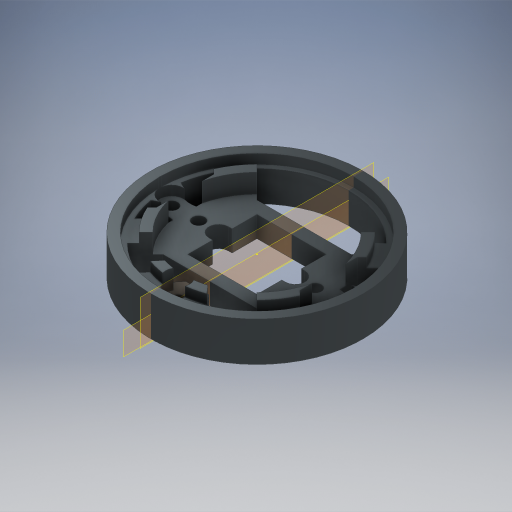
# Autodesk Inventor part: omv_centre
Saved by Autodesk Inventor 2023 (Build 270158000, 158)
## iProperties
Created: 2024-12-20
Part Number: omv_centre
Material: Типовые
Document SubType Name: Modeling
Designer: Ivan
Density: 1 g/cm^3
Appearance: Чугун серый
Mass: 9.16198 g
Surface Area: 75.1348 cm^2
Volume: 9.16198 cm^3
Author: Ivan
Autodesk Inventor part; units mm, degrees
ref_plane "XZ Plane" through (0, 0, 0) normal (0, 1, 0) x (-1, 0, 0)
ref_plane "XY Plane" through (0, 0, 0) normal (0, 0, 1) x (1, 0, 0)
sketch "Эскиз3" plane through (0, 0, 0) normal (0, 1, 0) x (-1, 0, 0)
  circle A0 centre (0, 0) radius 7
  arc A1 (-1.5597, 7.5914) -> (1.5597, 7.5914) centre (0, 0) ccw
  line L0 (1.4, 8.3) -> (1.4, 7.7873)
  arc A2 (1.4, 7.7873) -> (1.5597, 7.5914) centre (1.6, 7.7873) ccw
  arc A3 (1.4, 8.3) -> (1.2, 8.5) centre (1.2, 8.3) ccw
  line L1 (-1.2, 8.5) -> (1.2, 8.5)
  arc A4 (-1.2, 8.5) -> (-1.4, 8.3) centre (-1.2, 8.3) ccw
  line L2 (-1.4, 7.7873) -> (-1.4, 8.3)
  arc A5 (-1.5597, 7.5914) -> (-1.4, 7.7873) centre (-1.6, 7.7873) ccw
  line L3 (8.5, 7.5) -> (8.5, 1.9)
  arc A6 (8.5, 7.5) -> (7.5, 8.5) centre (7.5, 7.5) ccw
  line L4 (1.6, 8.5) -> (7.5, 8.5)
  line L5 (8.5, -1.9) -> (8.5, -7.5)
  arc A7 (7.5, -8.5) -> (8.5, -7.5) centre (7.5, -7.5) ccw
  line L6 (7.5, -8.5) -> (-7.5, -8.5)
  arc A8 (-8.5, -7.5) -> (-7.5, -8.5) centre (-7.5, -7.5) ccw
  line L7 (-8.5, -7.5) -> (-8.5, -1.9)
  line L8 (-7.5, 8.5) -> (-1.6, 8.5)
  arc A9 (-7.5, 8.5) -> (-8.5, 7.5) centre (-7.5, 7.5) ccw
  line L9 (-8.5, 1.9) -> (-8.5, 7.5)
  line L10 (-1.2, 8.5) -> (-1.6, 8.5)
  line L11 (1.6, 8.5) -> (1.2, 8.5)
  circle A10 centre (15.24, 0) radius 1.5
  circle A11 centre (-15.24, 0) radius 1.5
  arc A12 (-10, 1.9) -> (-10, -1.9) centre (-10, 0) ccw
  arc A13 (10, -1.9) -> (10, 1.9) centre (10, 0) ccw
  line L12 (8.5, 1.9) -> (10, 1.9)
  line L13 (10, -1.9) -> (8.5, -1.9)
  line L14 (-10, 1.9) -> (-8.5, 1.9)
  line L15 (-8.5, -1.9) -> (-10, -1.9)
  constraints: 32 end point, 22 point on circle, 14 centre point
sketch "Эскиз4" plane through (0, 0, 0) normal (0, 1, 0) x (-1, 0, 0)
  circle A0 centre (0, 0) radius 29
  circle A1 centre (0, 0) radius 26.45
  circle A2 centre (0, 0) radius 23.95
  circle A3 centre (0, 0) radius 31.5
  line L0 (-9.05, 2.55) -> (-9.05, 9.05)
  line L1 (-9.05, 9.05) -> (9.05, 9.05)
  line L2 (9.05, 9.05) -> (9.05, 2.55)
  line L3 (-9.05, -2.55) -> (-9.05, -9.05)
  line L4 (-9.05, -9.05) -> (9.05, -9.05)
  line L5 (9.05, -9.05) -> (9.05, -2.55)
  line L6 (-1.2, 8.5) -> (1.2, 8.5) projected
  line L7 (0, 8.5) -> (0, 9.05) construction
  line L8 (8.5, 7.5) -> (8.5, 1.9) projected
  line L9 (-8.5, 1.9) -> (-8.5, 7.5) projected
  line L10 (7.5, -8.5) -> (-7.5, -8.5) projected
  line L11 (8.5, 1.9) -> (10, 1.9) projected
  line L12 (9.05, 2.55) -> (10, 2.55)
  line L13 (9.05, -2.55) -> (10, -2.55)
  line L14 (-9.05, -2.55) -> (-10, -2.55)
  line L15 (-9.05, 2.55) -> (-10, 2.55)
  line L16 (10, 1.9) -> (10, 2.55) construction
  line L17 (10, 2.55) -> (10, -2.55) construction
  line L18 (-10, 2.55) -> (-10, -2.55) construction
  arc A4 (10, -2.55) -> (10, 2.55) centre (10, 0) ccw
  arc A5 (-10, 2.55) -> (-10, -2.55) centre (-10, 0) ccw
  circle A6 centre (-15.24, 0) radius 1.5 construction
  circle A7 centre (15.24, 0) radius 1.5 construction
  circle A8 centre (-15.24, 0) radius 1.6
  circle A9 centre (15.24, 0) radius 1.6
  line L19 (-9.05, 9.05) -> (-16.9352, 16.9352)
  line L20 (-9.05, -9.05) -> (-16.9352, -16.9352)
  line L21 (9.05, -9.05) -> (16.9352, -16.9352)
  line L22 (9.05, 9.05) -> (16.9352, 16.9352)
  line L23 (44.1, 0) -> (-44.1, 0) projected
  circle A10 centre (15.24, 0) radius 3.5 construction
  circle A11 centre (-15.24, 0) radius 3.5 construction
  line L24 (-18.74, 7.5) -> (-18.74, -7.5)
  line L25 (18.74, 7.5) -> (18.74, -7.5)
  line L26 (-18.74, 7.5) -> (-21.5955, 10.3555)
  line L27 (-18.74, -7.5) -> (-21.5955, -10.3555)
  line L28 (18.74, 7.5) -> (21.5955, 10.3555)
  line L29 (18.74, -7.5) -> (21.5955, -10.3555)
  line L30 (-12.28, 12.28) -> (12.28, 12.28)
  line L31 (-12.28, -12.28) -> (12.28, -12.28)
  point P0 (-16.84, 0)
  point P1 (16.84, 0)
  point P2 (18.74, 0)
  point P3 (-18.74, 0)
  dimension "d11" = 3.2
  dimension "d16" = 7
  dimension "d1" = 58
  dimension "d3" = 2.55
  dimension "d4" = 2.5
  dimension "d5" = 2.5
  dimension "d6" = 0.55
  dimension "d7" = 0.55
  dimension "d8" = 0.55
  dimension "d9" = 0.65
  dimension "d10" = 0.55
  dimension "d13" = 135
  dimension "d14" = 135
  dimension "d17" = 135
  dimension "d18" = 15
  dimension "d19" = 9.69
  dimension "d20" = 3.23
  dimension "d21" = 3.23
  constraints: 52 end point, 11 perpendicular, 8 coincident, 7 equal length, 6 midpoint, 6 point on line, 6 vertical, 5 centre point, 5 parallel, 4 horizontal alignment, 4 point on circle, 2 collinear, 2 horizontal, 18 other
  measures "d1" diameter of A0
  measures "d3" radial gap between concentric circles of A0 A1
  measures "d5" radial gap between concentric circles of A3 A0
  measures "d6" distance between parallel lines of L1 L6
  measures "d7" distance between parallel lines of L2 L8
  measures "d8" distance between parallel lines of L4 L10
  measures "d9" distance from line of L2.end L11
  measures "d10" distance between parallel lines of L9 L0
  measures "d13" angle of L22 L1
  measures "d14" angle of L19 L1
  measures "d17" angle of L28 L25
  measures "d18" distance of L24.start L24.end
  measures "d19" distance from line of L0 point (-18.74, 0)
  measures "d20" distance between parallel lines of L1 L30
  measures "d21" distance between parallel lines of L4 L31
extrude "Выдавливание1" add sketch "Эскиз4" along normal blind 5.5 contours L23 A3 A0 | A0 L23 A3 | L23 A2 A1 | A1 L23 A2 | L28 L25 L23 A9 A4 L12 L2 L22 A2 | A2 L21 L5 L13 A4 L23 A9 L25 L29 | A2 L19 L0 L15 A5 L23 A8 L24 L26 | L27 L24 L23 A8 A5 L14 L3 L20 A2 | L22 L1 L19 L30 | L31 L20 L4 L21
extrude "Выдавливание2" add sketch "Эскиз4" along normal blind 3.5 contours L23 A1 A0 | A0 L23 A1
chamfer "Фаска1" distance 4 angle 45 1 edges at (31.5, 0, 0)
sketch "Эскиз6" plane through (0, 0, 0) normal (0, -1, 0) x (1, 0, 0)
  circle A0 centre (-0.1305, 20.6127) radius 2.1 projected
  point P0 (0, 0)
sketch "Эскиз7" plane through (0, 0, 0) normal (0, -1, 0) x (1, 0, 0)
  circle A0 centre (-0.1305, 20.6127) radius 2.1 construction
  circle A1 centre (-0.1305, 20.6127) radius 1.6
  circle A2 centre (0, 0) radius 23.95 projected
  arc A3 (16.9352, 16.9352) -> (-16.9352, 16.9352) centre (0, 0) ccw projected
  line L0 (-8.9159, 22.2286) -> (-3.9, 17.2127)
  line L1 (-3.9, 17.2127) -> (3.9, 17.2127)
  line L2 (3.9, 17.2127) -> (8.9159, 22.2286)
  circle A4 centre (-0.1305, 20.6127) radius 3.4 construction
  point P0 (8.9159, 22.2286)
  dimension "d33" = 3.2
  dimension "d34" = 135
  dimension "d35" = 135
  dimension "d36" = 6.8
  dimension "d37" = 7.8
  constraints: 6 end point, 2 centre point, 2 coincident, 2 point on circle, 1 horizontal, 1 perpendicular, 1 tangent
  measures "d33" diameter of A1
  measures "d34" angle of L0 L1
  measures "d35" angle of L2 L1
  measures "d36" diameter of A4
  measures "d37" distance of L0.end L1.end
extrude "Выдавливание3" add sketch "Эскиз7" against normal up to surface (5.5 mm away) contours L2 L1 L0 A2 picked at (-5.7854, 20.9857)
sketch "Эскиз8" plane through (0, 0, 0) normal (0, -1, 0) x (1, 0, 0)
  circle A0 centre (14.6021, 5.1056) radius 2.1 projected
  circle A1 centre (-14.8609, 5.1034) radius 2.1 projected
  point P0 (0, 0)
sketch "Эскиз9" plane through (0, 0, 0) normal (0, -1, 0) x (1, 0, 0)
  circle A0 centre (-14.8609, 5.1034) radius 1.397 projected
  circle A1 centre (14.6031, 5.1142) radius 1.397 projected
  point P0 (0, 0)
sketch "Эскиз11" plane through (0, 0, 0) normal (0, -1, 0) x (1, 0, 0)
  circle A0 centre (15.24, 0) radius 1.6 projected
  circle A1 centre (15.24, 0) radius 3
  point P0 (0, 0)
  dimension "d44" = 6
  constraints: 1 centre point, 1 coincident
  measures "d44" diameter of A1
sketch "Эскиз12" plane through (0, 0, 0) normal (0, -1, 0) x (1, 0, 0)
  circle A0 centre (22.0195, 0) radius 2 projected
  circle A1 centre (27.6855, 0) radius 1.6
  point P0 (0, 0)
  dimension "d50" = 3.2
  dimension "d51" = 5.666
  constraints: 1 centre point
  measures "d50" diameter of A1
  measures "d51" distance of A1.centre A0.centre
sketch "Эскиз13" plane through (0, 0, 0) normal (0, -1, 0) x (1, 0, 0)
  circle A0 centre (22.15, 0.1589) radius 1.6
  circle A1 centre (22.15, 0.1589) radius 3.1 construction
  arc A2 (21.5955, -10.3555) -> (21.5955, 10.3555) centre (0, 0) ccw projected
  line L0 (18.74, 7.5) -> (18.74, -7.5) projected
  arc A3 (21.5955, -10.3555) -> (21.5955, 10.3555) centre (0, 0) ccw projected
  line L1 (18.74, 7.5) -> (18.74, -7.5) projected
  line L2 (21.5955, 10.3555) -> (18.74, 7.5) projected
  line L3 (18.74, -7.5) -> (21.5955, -10.3555) projected
  arc A4 (18.74, 3.2133) -> (23.5905, 4.1342) centre (20.1678, 8.9278) ccw
  arc A5 (23.6473, -3.7958) -> (18.74, -2.8941) centre (20.1678, -8.9278) ccw
  line L4 (0, 44.1) -> (0, -44.1) projected
  point P0 (11.24, 0)
  point P1 (18.74, -2.8941)
  point P2 (23.6473, -3.7958)
  point P3 (23.5905, 4.1342)
  point P4 (18.74, 3.2133)
  dimension "d45" = 3.2
  dimension "d46" = 6.2
  dimension "d49" = 22.15
  constraints: 6 point on circle, 4 centre point, 4 point on line, 3 coincident, 2 midpoint, 2 tangent
  measures "d45" diameter of A0
  measures "d46" diameter of A1
  measures "d49" distance from line of L4 point (22.15, 0.159)
extrude "Выдавливание5" add sketch "Эскиз13" against normal up to surface (5.5 mm away) contours A5 L0 A4 A2
ref_plane "РабПлоскость1" through (0, 0, 9.05) normal (1, 0, 0) x (0, 0, -1)
mirror "Зеркальное отражение2" about plane through (0, 0, 9.05) normal (1, 0, 0) of "Выдавливание5"
sketch "Эскиз14" plane through (0, 5.5, 0) normal (0, 1, 0) x (1, 0, 0)
  line L0 (3.9, -17.2127) -> (8.9159, -22.2286) projected
  line L1 (-8.9159, -22.2286) -> (-3.9, -17.2127) projected
  arc A0 (-16.9352, -16.9352) -> (-8.9159, -22.2286) centre (0, 0) ccw projected
  arc A1 (8.9159, -22.2286) -> (16.9352, -16.9352) centre (0, 0) ccw projected
  circle A2 centre (0, 0) radius 23.95
  line L2 (-8.9159, -22.2286) -> (-3.1305, -15.4166)
  line L3 (-3.1305, -15.4166) -> (2.8695, -15.4166)
  line L4 (3.9, -17.2127) -> (8.9159, -22.2286) projected
  line L5 (2.8695, -15.4166) -> (8.9159, -22.2286)
  line L6 (-3.9, -17.2127) -> (3.9, -17.2127) projected
  line L7 (-3.9, -17.2127) -> (3.9, -17.2127)
  line L8 (-8.9159, -22.2286) -> (-3.9, -17.2127) projected
  line L9 (-3.9, -17.2127) -> (3.9, -17.2127) projected
  line L10 (-3.9, -17.2127) -> (3.9, -17.2127)
  constraints: 10 end point, 3 point on circle, 1 centre point, 1 collinear, 1 horizontal, 2 other
extrude "Выдавливание6" add sketch "Эскиз14" against normal up to surface (5.5 mm away) contours L6 L1 L2 L3 L5 L0
sketch "Эскиз15" plane through (0, 5.5, 0) normal (0, 1, 0) x (1, 0, 0)
  point P0 (0, 0)
sketch "Эскиз16" plane through (0, 5.5, 0) normal (0, 1, 0) x (1, 0, 0)
  circle A0 centre (0, 0) radius 29 projected
  circle A1 centre (0, 0) radius 26.45 projected
extrude "Выдавливание7" add sketch "Эскиз16" against normal up to surface (2 mm away)
sketch "Эскиз17" plane through (0, 5.5, 0) normal (0, 1, 0) x (1, 0, 0)
  circle A0 centre (0, 0) radius 21.75
  circle A1 centre (0, 0) radius 25.25
  circle A2 centre (0, 0) radius 31.5 projected
  arc A3 (-21.5955, 10.3555) -> (-23.6473, 3.7958) centre (0, 0) ccw projected
  line L0 (-21.5955, 10.3555) -> (-18.74, 7.5) projected
  line L1 (-18.74, 7.5) -> (-18.74, 2.8941) projected
  arc A4 (-23.6473, 3.7958) -> (-18.74, 2.8941) centre (-20.1678, 8.9278) ccw projected
  circle A5 centre (-22.15, -0.1589) radius 1.6 projected
  arc A6 (21.5955, -10.3555) -> (23.5905, -4.1342) centre (0, 0) ccw projected
  line L2 (21.5955, -10.3555) -> (18.74, -7.5) projected
  line L3 (18.74, -7.5) -> (18.74, -3.2133) projected
  arc A7 (23.5905, -4.1342) -> (18.74, -3.2133) centre (20.1678, -8.9278) ccw projected
  circle A8 centre (22.15, -0.1589) radius 1.6 projected
  circle A9 centre (-0.1305, -20.6127) radius 1.6 projected
  arc A10 (18.74, 2.8941) -> (23.6473, 3.7958) centre (20.1678, 8.9278) ccw projected
  line L4 (18.74, 2.8941) -> (18.74, 7.5) projected
  line L5 (18.74, 7.5) -> (21.5955, 10.3555) projected
  arc A11 (23.6473, 3.7958) -> (21.5955, 10.3555) centre (0, 0) ccw projected
  arc A12 (-18.74, -3.2133) -> (-23.5905, -4.1342) centre (-20.1678, -8.9278) ccw projected
  line L6 (-18.74, -3.2133) -> (-18.74, -7.5) projected
  line L7 (-18.74, -7.5) -> (-21.5955, -10.3555) projected
  arc A13 (-23.5905, -4.1342) -> (-21.5955, -10.3555) centre (0, 0) ccw projected
  line L8 (-16.9352, -16.9352) -> (-12.28, -12.28) projected
  line L9 (-12.28, -12.28) -> (12.28, -12.28) projected
  line L10 (12.28, -12.28) -> (16.9352, -16.9352) projected
  arc A14 (8.9159, -22.2286) -> (16.9352, -16.9352) centre (0, 0) ccw projected
  line L11 (8.9159, -22.2286) -> (2.8695, -15.4166) projected
  line L12 (2.8695, -15.4166) -> (-3.1305, -15.4166) projected
  line L13 (-3.1305, -15.4166) -> (-8.9159, -22.2286) projected
  arc A15 (-16.9352, -16.9352) -> (-8.9159, -22.2286) centre (0, 0) ccw projected
  circle A16 centre (-15.24, 0) radius 1.6 projected
  circle A17 centre (15.24, 0) radius 1.6 projected
  arc A18 (16.9352, 16.9352) -> (-16.9352, 16.9352) centre (0, 0) ccw projected
  line L14 (16.9352, 16.9352) -> (12.28, 12.28) projected
  line L15 (12.28, 12.28) -> (-12.28, 12.28) projected
  line L16 (-12.28, 12.28) -> (-16.9352, 16.9352) projected
  line L17 (-9.05, -9.05) -> (-9.05, -2.55) projected
  line L18 (-9.05, -2.55) -> (-10, -2.55) projected
  arc A19 (-10, 2.55) -> (-10, -2.55) centre (-10, 0) ccw projected
  line L19 (-10, 2.55) -> (-9.05, 2.55) projected
  line L20 (-9.05, 2.55) -> (-9.05, 9.05) projected
  line L21 (-9.05, 9.05) -> (9.05, 9.05) projected
  line L22 (9.05, 9.05) -> (9.05, 2.55) projected
  line L23 (9.05, 2.55) -> (10, 2.55) projected
  arc A20 (10, -2.55) -> (10, 2.55) centre (10, 0) ccw projected
  line L24 (10, -2.55) -> (9.05, -2.55) projected
  line L25 (9.05, -2.55) -> (9.05, -9.05) projected
  line L26 (9.05, -9.05) -> (-9.05, -9.05) projected
  circle A21 centre (0, 0) radius 27.75
  circle A22 centre (0, 0) radius 19.25
  circle A23 centre (-22.15, -0.1589) radius 3.125
  circle A24 centre (22.15, -0.1589) radius 3.125
  circle A25 centre (-0.1305, -20.6127) radius 1.6 projected
  circle A26 centre (-0.1305, -20.6127) radius 3.125
  point P0 (25.2488, 0.2448)
  point P1 (25.2427, -0.607)
  point P2 (-25.2427, -0.607)
  point P3 (-25.2488, 0.2448)
  point P4 (-18.7899, 7.5499)
  point P5 (-13.6118, 13.6118)
  point P6 (13.6118, 13.6118)
  point P7 (18.7899, 7.5499)
  point P8 (21.8021, 2.9467)
  point P9 (-21.8021, 2.9467)
  point P10 (18.7899, -7.5499)
  point P11 (13.6118, -13.6118)
  point P12 (7.3541, -20.469)
  point P13 (-7.4057, -20.4504)
  point P14 (-13.6118, -13.6118)
  point P15 (-18.7899, -7.5499)
  point P16 (-21.7759, -3.2614)
  point P17 (21.7759, -3.2614)
  point P18 (5.5473, -18.4334)
  point P19 (2.59, -19.075)
  point P20 (-2.8313, -19.0407)
  point P21 (-5.6628, -18.3982)
  point P22 (18.74, 4.4017)
  point P23 (19.0407, 2.8307)
  point P24 (21.1729, 2.8094)
  point P25 (-21.1729, 2.8094)
  point P26 (-19.0407, 2.8307)
  point P27 (-18.74, 4.4017)
  point P28 (19.2268, 0.9458)
  point P29 (19.2112, -1.2215)
  point P30 (-19.2268, 0.9458)
  point P31 (-19.2112, -1.2215)
  point P32 (-18.74, -4.4017)
  point P33 (-18.9894, -3.1567)
  point P34 (-21.1532, -3.1206)
  point P35 (21.1532, -3.1206)
  point P36 (18.9894, -3.1567)
  point P37 (18.74, -4.4017)
  dimension "d56" = 43.5
  dimension "d57" = 50.5
  dimension "d58" = 3.5
  dimension "d59" = 2.5
  dimension "d60" = 2.5
  dimension "d61" = 6.25
  dimension "d62" = 6.25
  dimension "d65" = 6.25
  constraints: 7 coincident, 6 centre point, 2 other
  measures "d56" diameter of A0
  measures "d57" diameter of A1
  measures "d58" radial gap between concentric circles of A1 A0
  measures "d59" radial gap between concentric circles of A21 A1
  measures "d61" diameter of A23
  measures "d62" diameter of A24
  measures "d65" diameter of A26
extrude "Выдавливание8" add sketch "Эскиз17" along normal blind 2.5 contours A10 A11 L5 A0 L14 A18 L16 L0 A3 A4 A23 A1 A24 | A24 A1 A23 A12 A13 L7 A0 L8 A15 L13 A26 L11 A14 L10 L2 A6 A7 | L5 L4 A22 L14 A0 | A0 L10 A22 L3 L2 | L16 A22 L1 L0 A0 | A0 A26 A22 L11 | A0 L13 A22 A26 | L7 L6 A22 L8 A0 | A21
sketch "Эскиз18" plane through (0, 8, 0) normal (0, 1, 0) x (1, 0, 0)
  circle A0 centre (0, 0) radius 19.25 projected
  circle A1 centre (0, 0) radius 21.75 projected
  circle A2 centre (0, 0) radius 27.75 projected
  circle A3 centre (0, 0) radius 25.25
  circle A4 centre (0, 0) radius 27.75 projected
  arc A5 (21.7759, -3.2614) -> (21.8021, 2.9467) centre (22.15, -0.1589) ccw projected
  arc A6 (23.5905, -4.1342) -> (21.7759, -3.2614) centre (20.1678, -8.9278) ccw projected
  arc A7 (13.6118, -13.6118) -> (18.74, -4.4017) centre (0, 0) ccw projected
  arc A8 (2.59, -19.075) -> (5.5473, -18.4334) centre (0, 0) ccw projected
  arc A9 (-5.6628, -18.3982) -> (-2.8313, -19.0407) centre (0, 0) ccw projected
  arc A10 (-21.7759, -3.2614) -> (-23.5905, -4.1342) centre (-20.1678, -8.9278) ccw projected
  arc A11 (-21.8021, 2.9467) -> (-21.7759, -3.2614) centre (-22.15, -0.1589) ccw projected
  arc A12 (-23.6473, 3.7958) -> (-21.8021, 2.9467) centre (-20.1678, 8.9278) ccw projected
  line L0 (-13.6118, 13.6118) -> (-16.9352, 16.9352) projected
  line L1 (16.9352, 16.9352) -> (13.6118, 13.6118) projected
  arc A13 (21.8021, 2.9467) -> (23.6473, 3.7958) centre (20.1678, 8.9278) ccw projected
  arc A14 (21.5955, -10.3555) -> (23.5905, -4.1342) centre (0, 0) ccw projected
  line L2 (21.5955, -10.3555) -> (18.74, -7.5) projected
  line L3 (18.74, -7.5) -> (18.74, -4.4017) projected
  line L4 (13.6118, -13.6118) -> (16.9352, -16.9352) projected
  arc A15 (8.9159, -22.2286) -> (16.9352, -16.9352) centre (0, 0) ccw projected
  line L5 (8.9159, -22.2286) -> (5.5473, -18.4334) projected
  arc A16 (-2.8313, -19.0407) -> (2.59, -19.075) centre (-0.1305, -20.6127) ccw projected
  line L6 (-5.6628, -18.3982) -> (-8.9159, -22.2286) projected
  arc A17 (-16.9352, -16.9352) -> (-8.9159, -22.2286) centre (0, 0) ccw projected
  line L7 (-16.9352, -16.9352) -> (-13.6118, -13.6118) projected
  arc A18 (-18.74, -4.4017) -> (-13.6118, -13.6118) centre (0, 0) ccw projected
  line L8 (-18.74, -4.4017) -> (-18.74, -7.5) projected
  line L9 (-18.74, -7.5) -> (-21.5955, -10.3555) projected
  arc A19 (-23.5905, -4.1342) -> (-21.5955, -10.3555) centre (0, 0) ccw projected
  arc A20 (-21.5955, 10.3555) -> (-23.6473, 3.7958) centre (0, 0) ccw projected
  line L10 (-21.5955, 10.3555) -> (-18.74, 7.5) projected
  line L11 (-18.74, 7.5) -> (-18.74, 4.4017) projected
  arc A21 (-13.6118, 13.6118) -> (-18.74, 4.4017) centre (0, 0) ccw projected
  arc A22 (16.9352, 16.9352) -> (-16.9352, 16.9352) centre (0, 0) ccw projected
  arc A23 (18.74, 4.4017) -> (13.6118, 13.6118) centre (0, 0) ccw projected
  line L12 (18.74, 4.4017) -> (18.74, 7.5) projected
  line L13 (18.74, 7.5) -> (21.5955, 10.3555) projected
  arc A24 (23.6473, 3.7958) -> (21.5955, 10.3555) centre (0, 0) ccw projected
  point P0 (15.3796, 15.3796)
  point P1 (-15.3796, 15.3796)
  point P2 (-25.2427, -0.607)
  point P3 (-25.2488, 0.2448)
  point P4 (25.2488, 0.2448)
  point P5 (25.2427, -0.607)
  point P6 (21.5578, 2.8853)
  point P7 (21.5143, -3.1936)
  point P8 (-21.5578, 2.8853)
  point P9 (-21.5143, -3.1936)
  point P10 (-5.6628, -18.3982)
  point P11 (13.6118, -13.6118)
  point P12 (-18.74, -4.4017)
  point P13 (2.59, -19.075)
  point P14 (-2.8313, -19.0407)
  point P15 (18.74, 4.4017)
  point P16 (18.74, -4.4017)
  point P17 (-19.936, 8.696)
  point P18 (-19.936, -8.696)
  point P19 (-15.3796, -15.3796)
  point P20 (-7.4057, -20.4504)
  point P21 (-3.1193, -21.5252)
  point P22 (2.8465, -21.5629)
  point P23 (7.3541, -20.469)
  point P24 (15.3796, -15.3796)
  point P25 (19.936, -8.696)
  point P26 (19.936, 8.696)
  dimension "d66" = 2.5
  constraints: 1 centre point, 1 coincident
  measures "d66" radial gap between concentric circles of A3 A2
extrude "Выдавливание9" add sketch "Эскиз18" along normal blind 2.5 contours A0 L1 A1 L13 L12 | L3 L2 A1 L4 A0 | A0 L11 L10 A1 L0 | L5 A1 A16 A0 | A0 L7 A1 L9 L8 | A16 A1 L6 A0 | A2
sketch "Эскиз19" plane through (0, 5.5, 0) normal (0, 1, 0) x (1, 0, 0)
  circle A0 centre (0, 0) radius 27.75 projected
  circle A1 centre (0, 0) radius 31.5 projected
extrude "Выдавливание10" cut sketch "Эскиз19" against normal through all
equation "\"d5\" = d4"
equation "\"d7\" = d6"
equation "\"d8\" = d6"
equation "\"d10\" = d6"
equation "\"d20\" = 0.333333 * d19"
equation "\"d21\" = 0.333333 * d19"
equation "\"d35\" = d34"
equation "\"d60\" = d59"
